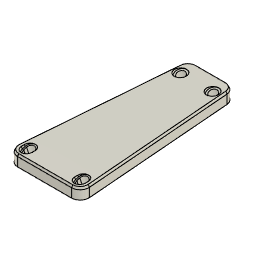
underseat-tray (Autodesk Fusion 360 design; units mm, degrees)
Autodesk Fusion 360 part; units mm, degrees
sketch "Sketch1" plane through (0, 0, 0) normal (0, 0, 1) x (1, 0, 0)
  circle A0 centre (-15.1, 66.4157) radius 3.6
  circle A1 centre (15.1, 66.4157) radius 3.6
  line L0 (-21.35, -67.8157) -> (-21.35, -65.0157)
  arc A2 (-21.35, -65.0157) -> (-28.55, -65.0157) centre (-24.95, -65.0157) ccw
  line L1 (-28.55, -65.0157) -> (-28.55, -67.8157)
  arc A3 (-28.55, -67.8157) -> (-21.35, -67.8157) centre (-24.95, -67.8157) ccw
  line L2 (-24.95, -67.8157) -> (-24.95, -65.0157) construction
  line L3 (28.55, -67.8157) -> (28.55, -65.0157)
  arc A4 (28.55, -65.0157) -> (21.35, -65.0157) centre (24.95, -65.0157) ccw
  line L4 (21.35, -65.0157) -> (21.35, -67.8157)
  arc A5 (21.35, -67.8157) -> (28.55, -67.8157) centre (24.95, -67.8157) ccw
  line L5 (24.95, -67.8157) -> (24.95, -65.0157) construction
  line L6 (21.35, -66.4157) -> (-21.35, -66.4157) construction
  line L7 (0, 0) -> (0, -66.4157) construction
  line L8 (0, 0) -> (0, 66.4157) construction
  line L9 (-11.5, 66.4157) -> (11.5, 66.4157) construction
  line L10 (11.5, 62.5719) -> (11.5, 70.0303) construction
  line L11 (-11.5, 69.0679) -> (-11.5, 63.414) construction
  line L12 (-21.5, 77.0157) -> (21.5, 77.0157)
  line L13 (21.5, 77.0157) -> (34, -79.4157)
  line L14 (34, -79.4157) -> (-34, -79.4157)
  line L15 (-34, -79.4157) -> (-21.5, 77.0157)
  line L16 (-30.5341, -76.2157) -> (-18.5455, 73.8157)
  line L17 (-18.5455, 73.8157) -> (18.5455, 73.8157)
  line L18 (18.5455, 73.8157) -> (30.5341, -76.2157)
  line L19 (30.5341, -76.2157) -> (-30.5341, -76.2157)
  line L20 (-23.194, 55.8157) -> (23.194, 55.8157)
  line L21 (-32.0023, -54.4157) -> (32.0023, -54.4157)
  line L22 (-23.4497, 52.6157) -> (23.4497, 52.6157)
  line L23 (-31.7466, -51.2157) -> (31.7466, -51.2157)
  point P0 (-24.95, -66.4157)
  point P1 (24.95, -66.4157)
  dimension "d1" = 7.2
  dimension "d2" = 7.2
  dimension "d3" = 7.2
  dimension "d4" = 7.2
  dimension "d5" = 10
  dimension "d6" = 10
  dimension "d8" = 42.7
  dimension "d9" = 23
  dimension "d10" = 124.6
  dimension "d11" = 43
  dimension "d12" = 21.5
  dimension "d13" = 68
  dimension "d14" = 34
  dimension "d15" = 7
  dimension "d16" = 8
  dimension "d17" = 3.2
  dimension "d19" = 7
  dimension "d20" = 7
  dimension "d23" = 3.2
  dimension "d24" = 3.2
  constraint tangent L0 A2
  constraint tangent A2 L1
  constraint parallel L0 L1
  constraint tangent L1 A3
  constraint tangent L0 A3
  constraint vertical L2
  constraint midpoint L2 P0
  constraint tangent L3 A4
  constraint tangent A4 L4
  constraint parallel L3 L4
  constraint tangent L4 A5
  constraint tangent L3 A5
  constraint parallel L0 L5
  constraint midpoint L5 P1
  constraint midpoint L4 L6.start
  constraint midpoint L0 L6.end
  constraint horizontal L6
  constraint coincident L7.start L8.start
  constraint midpoint L6 L7.end
  constraint parallel L7 L8
  constraint vertical L8
  constraint coincident A0 L9.start
  constraint coincident A1 L9.end
  constraint horizontal L9
  constraint midpoint L8.end L9
  constraint equal L7 L8
  constraint vertical L10
  constraint parallel L10 L11
  constraint coincident L9.start L11
  constraint coincident L9.end L10
  constraint tangent A1 L10
  constraint tangent A0 L11
  constraint horizontal L12
  constraint parallel L12 L14
  constraint coincident L15 L20.start
  constraint coincident L13 L20.end
  constraint perpendicular L8 L20
  constraint coincident L15 L21.start
  constraint coincident L13 L21.end
  constraint parallel L20 L21
  constraint coincident L15 L22.start
  constraint coincident L13 L22.end
  constraint horizontal L22
  constraint coincident L15 L23.start
  constraint coincident L13 L23.end
  constraint perpendicular L7 L23
  measures "d1" diameter of A0
  measures "d2" diameter of A1
  measures "d3" distance of L0 L1
  measures "d4" distance of L3 L4
  measures "d8" distance of L6.start L6.end
  measures "d9" distance of L9.start L9.end
  measures "d10" distance of A1 A4
  measures "d11" distance of L12.start L12.end
  measures "d12" horizontal distance of L7.start L12.end
  measures "d13" distance of L13.end L14.end
  measures "d14" horizontal distance of L7.start L13.end
  measures "d15" distance of A1 L12
  measures "d16" distance of A5 L14
  measures "d19" distance of A1 L20
  measures "d20" distance of A4 L21
  measures "d23" distance of L21 L23
  measures "d24" distance of L20 L22
extrude "Extrude1" add sketch "Sketch1" along normal blind 8 contours A0 | A1 | L0 A2 L1 A3 | L3 A4 L4 A5 | L12 L13 L15 L16 L17 L18 L20 | L15 L16 L20 L22 | L13 L18 L20 L22 | L15 L16 L22 L23 | L16 L17 L18 L20 | L13 L18 L22 L23 | L15 L16 L21 L23 | L13 L18 L21 L23 | L13 L14 L15 L16 L18 L19 L21 | L16 L18 L19 L21
extrude "Extrude5" add sketch "Sketch1" along normal blind 2.4 from surface at 8 contours A0 | A1 | L0 A2 L1 A3 | L3 A4 L4 A5 | L12 L13 L15 L16 L17 L18 L20 | L15 L16 L20 L22 | L13 L18 L20 L22 | L15 L16 L22 L23 | L16 L18 L20 L22 | L16 L17 L18 L20 | L13 L18 L22 L23 | L15 L16 L21 L23 | L16 L18 L22 L23 | L13 L18 L21 L23 | L13 L14 L15 L16 L18 L19 L21 | L16 L18 L21 L23 | L16 L18 L19 L21
fillet "Fillet2" radius 8 4 edges at (-34, -79.4157, 5.2) (34, -79.4157, 5.2) (21.5, 77.0157, 5.2) (-21.5, 77.0157, 5.2)
chamfer "Chamfer3" distance 1 distance2 2 8 edges at (-27.6991, -0.5628, 10.4) (-31.2131, -76.8426, 10.4) (0, -79.4157, 10.4) (31.2131, -76.8426, 10.4) (27.6991, -0.5628, 10.4) (19.5406, 74.8935, 10.4) (0, 77.0157, 10.4) (-19.5406, 74.8935, 10.4) measured on face at (7.3628, -23.968, 10.4) measured on face at (-25.7019, -79.4073, 3.4667) measured on face at (7.3628, -23.968, 10.4) measured on face at (32.2925, -75.365, 3.4667) measured on face at (7.3628, -23.968, 10.4) measured on face at (20.0972, 74.326, 6.9333) measured on face at (7.3628, -23.968, 10.4) measured on face at (-20.8196, 73.3782, 3.4667)
sketch "Sketch3" plane through (0, 0, 0) normal (1, 0, 0) x (0, 1, 0)
  line L0 (66.4157, 0) -> (58.8029, 23.4298)
  line L1 (-66.4157, 0) -> (-75.3617, 27.5331)
  line L2 (-67.8157, 0) -> (-65.0157, 0)
  line L3 (70.0157, 0) -> (62.8157, 0)
  dimension "d47" = 72
  dimension "d50" = 72
  constraint midpoint L0.start L3
  constraint midpoint L1.start L2
  measures "d47" angle of L1 L2
  measures "d50" angle of L0 L3
ref_plane "WorkPlane1" through (0, 60.3722, 18.6001) normal (0, -0.309017, 0.951057) x (1, 0, 0)
sketch "Sketch4" plane through (0, 60.3722, 18.6001) normal (0, -0.309017, 0.951057) x (1, 0, 0)
  ellipse E0 centre (15.1, 0) end of major axis (18.7, 0) minor radius 3.4238
  ellipse E1 centre (-15.1, 0) end of major axis (-11.5, 0) minor radius 3.4238
  circle A0 centre (15.1, 0) radius 3.7
  circle A1 centre (-15.1, 0) radius 3.7
  dimension "d64" = 7.4
  dimension "d65" = 7.4
  constraint concentric E0 A0
  constraint concentric E1 A1
  measures "d64" diameter of A0
  measures "d65" diameter of A1
extrude "Extrude6" cut sketch "Sketch4" against normal through all contours E0 | E1 | A0 | A1
ref_plane "WorkPlane2" through (0, -74.6951, 25.4815) normal (0, -0.309017, 0.951057) x (1, 0, 0)
sketch "Sketch5" plane through (0, -74.6951, 25.4815) normal (0, -0.309017, 0.951057) x (1, 0, 0)
  line L0 (28.65, -1.4) -> (28.65, 1.4)
  arc A0 (28.65, 1.4) -> (21.25, 1.4) centre (24.95, 1.4) ccw
  line L1 (21.25, 1.4) -> (21.25, -1.4)
  arc A1 (21.25, -1.4) -> (28.65, -1.4) centre (24.95, -1.4) ccw
  line L2 (24.95, -1.4) -> (24.95, 1.4) construction
  line L3 (-21.25, -1.4) -> (-21.25, 1.4)
  arc A2 (-21.25, 1.4) -> (-28.65, 1.4) centre (-24.95, 1.4) ccw
  line L4 (-28.65, 1.4) -> (-28.65, -1.4)
  arc A3 (-28.65, -1.4) -> (-21.25, -1.4) centre (-24.95, -1.4) ccw
  line L5 (-24.95, -1.4) -> (-24.95, 1.4) construction
  point P0 (24.95, 0)
  point P1 (-24.95, 0)
  point P2 (24.95, 0)
  point P3 (-24.95, 0)
  dimension "d69" = 7.4
  dimension "d70" = 7.4
  dimension "d71" = 10.2
  dimension "d72" = 10.2
  constraint tangent L0 A0
  constraint tangent A0 L1
  constraint parallel L0 L1
  constraint tangent L1 A1
  constraint tangent L0 A1
  constraint vertical L2
  constraint coincident P2 P0
  constraint midpoint L2 P2
  constraint tangent L3 A2
  constraint tangent A2 L4
  constraint parallel L3 L4
  constraint tangent L4 A3
  constraint tangent L3 A3
  constraint parallel L0 L5
  constraint coincident P3 P1
  constraint midpoint L5 P3
  measures "d69" distance of L3 L4
  measures "d70" distance of L0 L1
extrude "Extrude7" cut sketch "Sketch5" against normal through all
sketch "Sketch6" plane through (0, 60.3722, 18.6001) normal (0, -0.309017, 0.951057) x (1, 0, 0)
  ellipse E0 centre (-15.1, 0) end of major axis (-11.5, 0) minor radius 3.4238
  ellipse E1 centre (15.1, 0) end of major axis (18.7, 0) minor radius 3.4238
  circle A0 centre (-15.1, 0) radius 5.5
  circle A1 centre (15.1, 0) radius 5.5
  dimension "d75" = 11
  dimension "d76" = 11
  constraint concentric E0 A0
  constraint concentric E1 A1
  measures "d75" diameter of A0
  measures "d76" diameter of A1
extrude "Extrude8" cut sketch "Sketch6" against normal blind 10.603 contours E0 | E1 | A0 | A1
sketch "Sketch7" plane through (0, -74.6951, 25.4815) normal (0, -0.309017, 0.951057) x (1, 0, 0)
  arc A0 (-21.25, 1.4) -> (-28.65, 1.4) centre (-24.95, 1.4) ccw
  line L0 (-21.25, -1.4) -> (-21.25, 1.4)
  arc A1 (-28.65, -1.4) -> (-21.25, -1.4) centre (-24.95, -1.4) ccw
  line L1 (-28.65, 1.4) -> (-28.65, -1.4)
  arc A2 (28.65, 1.4) -> (21.25, 1.4) centre (24.95, 1.4) ccw
  line L2 (21.25, 1.4) -> (21.25, -1.4)
  arc A3 (21.25, -1.4) -> (28.65, -1.4) centre (24.95, -1.4) ccw
  line L3 (28.65, -1.4) -> (28.65, 1.4)
  line L4 (-19.95, -1.4) -> (-19.95, 1.4)
  arc A4 (-19.95, 1.4) -> (-29.95, 1.4) centre (-24.95, 1.4) ccw
  line L5 (-29.95, 1.4) -> (-29.95, -1.4)
  arc A5 (-29.95, -1.4) -> (-19.95, -1.4) centre (-24.95, -1.4) ccw
  line L6 (29.95, -1.4) -> (29.95, 1.4)
  arc A6 (29.95, 1.4) -> (19.95, 1.4) centre (24.95, 1.4) ccw
  line L7 (19.95, 1.4) -> (19.95, -1.4)
  arc A7 (19.95, -1.4) -> (29.95, -1.4) centre (24.95, -1.4) ccw
  dimension "d79" = 1.3
  dimension "d80" = 10
  dimension "d81" = 1.3
  measures "d80" distance of L4 L5
extrude "Extrude9" cut sketch "Sketch7" against normal blind 18.2266 contours A0 L0 A1 L1 | A2 L2 A3 L3 | L4 A4 L5 A5 | L6 A6 L7 A7
equation "d2 = d1"
equation "d12 = d11 / 2"
equation "d14 = d13 / 2"
equation "d17 = ( 0.4 * 8 ) * 1 mm"
equation "d23 = d17"
equation "d24 = d17"
equation "d47 = 90 deg - 18 deg"
equation "d50 = d47"
equation "d64 = d65"
equation "d70 = d69"
equation "d72 = d71"
equation "d76 = d75"
equation "d81 = d79"
